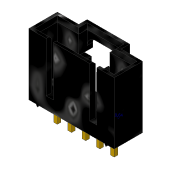
# Autodesk Inventor part: Molex_5
Saved by Autodesk Inventor 2017 (Build 210142000, 142)
## iProperties
Part Number: Molex_5
Material: Generisch
Document SubType Name: Modeling
Designer: David Merges
Density: 1 g/cm^3
Appearance: Schwarz
Author: David Merges
Autodesk Inventor part; units mm, degrees
ref_plane "YZ Plane" through (0, 0, 0) normal (1, 0, 0) x (0, 1, 0)
ref_plane "XZ Plane" through (0, 0, 0) normal (0, 1, 0) x (-1, 0, 0)
ref_plane "XY Plane" through (0, 0, 0) normal (0, 0, 1) x (1, 0, 0)
sketch "Skizze1" plane through (0, 0, 0) normal (0, 0, 1) x (1, 0, 0)
  line L0 (-12.705, -2.545) -> (2.545, -2.545)
  line L1 (2.545, -2.545) -> (2.545, 2.545)
  line L2 (2.545, 2.545) -> (-1.27, 2.545)
  line L3 (-1.27, 2.545) -> (-1.27, 4.055)
  line L4 (-1.27, 4.055) -> (-8.89, 4.055)
  line L5 (-8.89, 4.055) -> (-8.89, 2.545)
  line L6 (-8.89, 2.545) -> (-12.705, 2.545)
  line L7 (-12.705, 2.545) -> (-12.705, -2.545)
  line L8 (-7.87, 3.035) -> (-2.29, 3.035)
  line L9 (-2.29, 3.035) -> (-2.29, 1.525)
  line L10 (-2.29, 1.525) -> (1.525, 1.525)
  line L11 (1.525, 1.525) -> (1.525, -1.525)
  line L12 (1.525, -1.525) -> (-11.685, -1.525)
  line L13 (-11.685, -1.525) -> (-11.685, 1.525)
  line L14 (-11.685, 1.525) -> (-7.87, 1.525)
  line L15 (-7.87, 1.525) -> (-7.87, 3.035)
  line L16 (-11.685, 0) -> (-10.16, 0) construction
  line L17 (-10.16, 0) -> (0, 0) construction
  line L18 (0, 0) -> (1.525, 0) construction
  point P0 (0, -2.035)
  dimension "d0" = 1.02
  dimension "d1" = 3.05
  dimension "d3" = 7.62
  dimension "d4" = 6.6
  dimension "d5" = 1.525
  dimension "d6" = 10.16
  constraints: 38 end point, 12 perpendicular, 3 collinear, 2 horizontal, 2 midpoint, 2 point on line, 7 other
  measures "d0" distance between parallel lines of L4 L8
  measures "d1" distance between parallel lines of L12 L10
  measures "d3" distance between parallel lines of L3 L5
  measures "d4" distance between parallel lines of L4 L0
  measures "d5" distance from line of L11 L17.end
  measures "d6" distance of L16.end L17.end
extrude "Extrusion1" add sketch "Skizze1" along normal blind 3.8
sketch "Skizze2" plane through (0, 0, 0) normal (0, 0, -1) x (-1, 0, 0)
  line L0 (-2.545, -2.545) -> (-2.545, 2.545) projected
  line L1 (-2.545, 2.545) -> (1.27, 2.545) projected
  line L2 (-1.525, 1.525) -> (2.29, 1.525) projected
  line L3 (-1.525, -1.525) -> (-1.525, 1.525) projected
  line L4 (11.685, -1.525) -> (-1.525, -1.525) projected
  line L5 (12.705, -2.545) -> (-2.545, -2.545) projected
  line L6 (12.705, 2.545) -> (12.705, -2.545) projected
  line L7 (11.685, 1.525) -> (11.685, -1.525) projected
  line L8 (7.87, 1.525) -> (11.685, 1.525) projected
  line L9 (8.89, 2.545) -> (12.705, 2.545) projected
  line L10 (2.29, 1.525) -> (3.58, 1.525)
  line L11 (1.27, 2.545) -> (1.27, 4.055) projected
  line L12 (1.27, 2.545) -> (3.58, 2.545)
  line L13 (3.58, 2.545) -> (3.58, 1.525)
  line L14 (7.87, 1.525) -> (7.87, 3.035) projected
  line L15 (7.87, 1.525) -> (6.58, 1.525)
  line L16 (8.89, 2.545) -> (6.58, 2.545)
  line L17 (6.58, 2.545) -> (6.58, 1.525)
  point P0 (0, 0)
  dimension "d9" = 3
  constraints: 12 end point, 4 horizontal, 2 perpendicular, 1 collinear
  measures "d9" distance between parallel lines of L13 L17
extrude "Extrusion2" add sketch "Skizze2" along normal blind 5.09
sketch "Skizze3" plane through (0, 0, -5.09) normal (0, 0, -1) x (-1, 0, 0)
  line L0 (-2.545, 2.545) -> (-2.545, -2.545) projected
  line L1 (12.705, 2.545) -> (12.705, -2.545) projected
  line L2 (-2.545, -2.545) -> (12.705, -2.545)
  line L3 (12.705, -2.545) -> (12.705, 2.545)
  line L4 (12.705, 2.545) -> (-2.545, 2.545)
  line L5 (-2.545, 2.545) -> (-2.545, -2.545)
  point P0 (0, 0)
  constraints: 8 end point, 2 parallel, 1 horizontal, 1 perpendicular
extrude "Extrusion3" add sketch "Skizze3" along normal blind 2.16
sketch "Skizze4" plane through (-8.89, 4.055, 0) normal (0, 1, 0) x (1, 0, 0)
  line L0 (7.62, -3.8) -> (0, -3.8) construction
  line L1 (1.02, 0) -> (2.31, 0) projected
  line L2 (5.1, -2.3) -> (2.52, -2.3)
  line L3 (1.02, -0.8) -> (1.02, 0)
  line L4 (1.02, 0) -> (6.6, 0)
  line L5 (6.6, 0) -> (6.6, -0.8)
  arc A0 (5.1, -2.3) -> (6.6, -0.8) centre (5.1, -0.8) ccw
  arc A1 (1.02, -0.8) -> (2.52, -2.3) centre (2.52, -0.8) ccw
  line L6 (0, 0) -> (0, -3.8) construction
  line L7 (6.6, 0) -> (6.6, -3.8) construction
  line L8 (6.6, 0) -> (6.6, -3.8) construction
  line L9 (1.02, 0) -> (1.02, -3.8) construction
  line L10 (1.02, 0) -> (1.02, -3.8) construction
  point P0 (8.89, 0)
  dimension "d14" = 1.5
  dimension "d15" = 1.5
  constraints: 8 end point, 4 point on circle, 4 tangent, 2 centre point, 2 collinear, 2 parallel, 1 equal radius, 1 horizontal, 1 perpendicular, 1 point on line
  measures "d14" radius of A0
  measures "d15" distance between parallel lines of L0 L2
extrude "Extrusion4" cut sketch "Skizze4" against normal up to surface (1.02 mm away)
sketch "Skizze5" plane through (-12.705, -2.545, 3.8) normal (0, -1, 0) x (1, 0, 0)
  line L0 (0, -11.05) -> (1.2806, -11.05) construction
  line L1 (15.25, -11.05) -> (13.9694, -11.05) construction
  line L2 (1.2806, -11.05) -> (1.7194, -11.05)
  line L3 (1.7194, -11.05) -> (13.5306, -11.05) construction
  line L4 (13.5306, -11.05) -> (13.9694, -11.05)
  line L5 (13.5306, -11.05) -> (13.75, -11.43)
  line L6 (13.75, -11.43) -> (13.9694, -11.05)
  line L7 (1.7194, -11.05) -> (1.5, -11.43)
  line L8 (1.5, -11.43) -> (1.2806, -11.05)
  line L9 (15.25, -11.05) -> (15.25, 0) projected
  point P0 (12.705, -3.8)
  point P1 (0, -11.05)
  dimension "d18" = 0.38
  dimension "d19" = 1.5
  constraints: 18 end point, 5 equal length, 3 horizontal, 2 coincident, 1 collinear, 1 parallel, 1 point on line
  measures "d18" distance from line of L4 L5.end
  measures "d19" distance from line of L5.end L9
extrude "Extrusion5" add sketch "Skizze5" against normal up to surface (5.09 mm away)
sketch "Skizze6" plane through (0, 0, -5.09) normal (0, 0, 1) x (1, 0, 0)
  line L0 (-0.32, 0.32) -> (0.32, 0.32)
  line L1 (0.32, 0.32) -> (0.32, -0.32)
  line L2 (0.32, -0.32) -> (-0.32, -0.32)
  line L3 (-0.32, -0.32) -> (-0.32, 0.32)
  line L4 (0.32, -0.32) -> (-0.32, 0.32) construction
  point P0 (0, 0)
  point P1 (0, 0)
  dimension "d22" = 0.64
  constraints: 10 end point, 2 parallel, 2 perpendicular, 1 coincident, 1 horizontal, 1 midpoint
  measures "d22" distance of L0.start L0.end
extrude "Extrusion6" add sketch "Skizze6" along normal blind 6.1 and the other way blind 5.84
chamfer "Fase1" distance 0.2 angle 45 8 edges at (0, 0.32, 1.01) (0.32, 0, 1.01) (0, -0.32, 1.01) (-0.32, 0, 1.01) (0.32, 0, -10.93) (-0.32, 0, -10.93) (0, -0.32, -10.93) (0, 0.32, -10.93)
pattern_linear "Rechteckige Anordnung1" count 5 spacing 2.54 along (-1, 0, 0) of "Extrusion6", "Fase1"
sketch "Skizze8" plane through (0, 0, 3.8) normal (0, 0, 1) x (1, 0, 0)
  line L0 (1.525, -1.525) -> (-11.685, -1.525) construction
  line L1 (-12.705, -2.545) -> (2.545, -2.545) construction
  line L2 (-1.825, -2.035) -> (-8.335, -2.035) construction
  line L3 (-5.08, -2.545) -> (-5.08, -2.035) construction
  line L4 (-9.605, -1.525) -> (-8.335, -1.525)
  line L5 (-8.335, -1.525) -> (-8.335, -2.545)
  line L6 (-8.335, -2.545) -> (-9.605, -2.545)
  line L7 (-9.605, -2.545) -> (-9.605, -1.525)
  line L8 (-1.825, -1.525) -> (-0.555, -1.525)
  line L9 (-0.555, -1.525) -> (-0.555, -2.545)
  line L10 (-0.555, -2.545) -> (-1.825, -2.545)
  line L11 (-1.825, -2.545) -> (-1.825, -1.525)
  line L12 (-12.705, 2.545) -> (-12.705, -2.545) projected
  point P0 (0, 0)
  dimension "d33" = 1.27
  dimension "d34" = 3.1
  constraints: 21 end point, 4 midpoint, 4 parallel, 3 collinear, 3 perpendicular, 2 horizontal, 2 point on line
  measures "d33" distance between parallel lines of L5 L7
  measures "d34" distance between parallel lines of L7 L12
extrude "Extrusion7" cut sketch "Skizze8" against normal up to surface (8.89 mm away)
chamfer "Fase2" distance 0.51 angle 45 10 edges at (-11.685, 0, 3.8) (-10.645, -1.525, 3.8) (-9.7775, 1.525, 3.8) (-7.87, 2.28, 3.8) (-5.08, 3.035, 3.8) (-2.29, 2.28, 3.8) (-0.3825, 1.525, 3.8) (1.525, 0, 3.8) (0.485, -1.525, 3.8) (-5.08, -1.525, 3.8)
